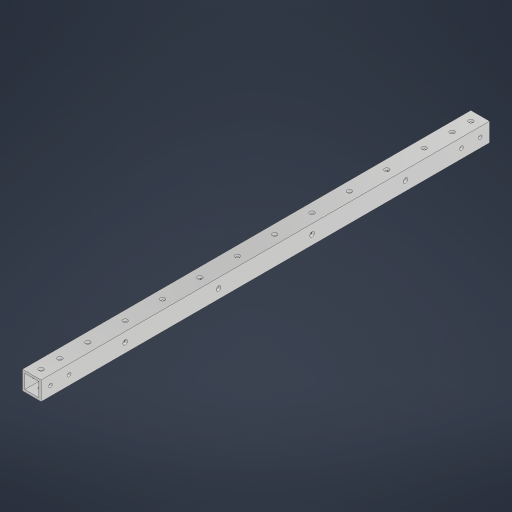
# Autodesk Inventor part: testRoboRescue_Chassis_Frame_widthBar
Saved by Autodesk Inventor 2023 (Build 270158000, 158)
## iProperties
Created: 2022-03-14
Part Number: testRoboRescue_Chassis_Frame_widthBar
Material: Aluminum 6061
Document SubType Name: Modeling
Designer: Nebil Oumer
Density: 2.7 g/cm^3
Appearance: Aluminum - Polished
Mass: 517.114 g
Surface Area: 1215.32 cm^2
Volume: 191.524 cm^3
Author: Nebil Oumer
Autodesk Inventor part; units mm, degrees
ref_plane "YZ Plane" through (0, 0, 0) normal (1, 0, 0) x (0, 1, 0)
ref_plane "XZ Plane" through (0, 0, 0) normal (0, 1, 0) x (-1, 0, 0)
ref_plane "XY Plane" through (0, 0, 0) normal (0, 0, 1) x (1, 0, 0)
sketch "Sketch1" plane through (0, 0, 0) normal (0, 0, 1) x (1, 0, 0)
  line L0 (0, 0) -> (25.4, 0)
  line L1 (25.4, 0) -> (25.4, 25.4)
  line L2 (25.4, 25.4) -> (0, 25.4)
  line L3 (0, 25.4) -> (0, 0)
  line L4 (3.175, 22.225) -> (22.225, 22.225)
  line L5 (22.225, 22.225) -> (22.225, 3.175)
  line L6 (22.225, 3.175) -> (3.175, 3.175)
  line L7 (3.175, 3.175) -> (3.175, 22.225)
  dimension "d0" = 25.4
  dimension "d1" = 25.4
  dimension "d2" = 3.175
  constraints: 16 end point, 4 parallel, 2 perpendicular, 1 horizontal, 3 other
  measures "d0" distance of L2.end L1.end
  measures "d1" distance of L1.end L0.end
  measures "d2" distance between parallel lines of L2 L4
extrude "Extrusion1" add sketch "Sketch1" along normal blind 609.6
sketch "Sketch2" plane through (0, 25.4, 0) normal (0, 1, 0) x (1, 0, 0)
  line L0 (25.4, 0) -> (25.4, -609.6) projected
  line L1 (25.4, -609.6) -> (0, -609.6) projected
  point P0 (0, 0)
  point P1 (12.7, -596.9)
  dimension "d12" = 12.7
  dimension "d13" = 12.7
  measures "d12" distance from line of L0 point (12.7, -596.9)
  measures "d13" distance from line of L1 point (12.7, -596.9)
hole "Hole1" at (12.7, 25.4, 596.9) direction (0, -1, 0) diameter 6.35 end through all
sketch "Sketch3" plane through (0, 25.4, 0) normal (0, 1, 0) x (1, 0, 0)
  line L0 (25.4, 0) -> (0, 0) projected
  line L1 (25.4, 0) -> (25.4, -609.6) projected
  point P0 (12.7, -12.7)
  dimension "d14" = 12.7
  dimension "d15" = 12.7
  measures "d14" distance from line of L0 point (12.7, -12.7)
  measures "d15" distance from line of L1 point (12.7, -12.7)
hole "Hole2" at (12.7, 25.4, 12.7) direction (0, -1, 0) diameter 6.35 end through all
pattern_linear "Rectangular Pattern1" count 2 spacing 25.4 along (0, 0, -1) count 2 spacing 25.4 along (0, 0, 1) of "Hole1", "Hole2"
sketch "Sketch4" plane through (25.4, 0, 0) normal (1, 0, 0) x (0, 0, -1)
  line L0 (0, 25.4) -> (-609.6, 25.4) projected
  line L1 (-609.6, 0) -> (-609.6, 25.4) projected
  line L2 (0, 0) -> (0, 25.4) projected
  point P0 (-596.9, 12.7)
  point P1 (-12.7, 12.7)
  dimension "d29" = 12.7
  dimension "d30" = 12.7
  dimension "d31" = 12.7
  dimension "d32" = 12.7
  measures "d29" distance from line of L0 point (-596.9, 12.7)
  measures "d30" distance from line of L1 point (-596.9, 12.7)
  measures "d31" distance from line of L2 point (-12.7, 12.7)
  measures "d32" distance from line of L0 point (-12.7, 12.7)
hole "Hole3" at (25.4, 12.7, 596.9) at (25.4, 12.7, 12.7) direction (-1, 0, 0) diameter 5.08 end through all
pattern_linear "Rectangular Pattern2" count 2 spacing 25.4 along (0, 0, -1) count 2 spacing 25.4 along (0, 0, 1) of "Hole3"
sketch "Sketch5" plane through (0, 25.4, 0) normal (0, 1, 0) x (1, 0, 0)
  line L0 (25.4, 0) -> (25.4, -609.6) projected
  circle A0 centre (12.7, -571.5) radius 3.175 projected
  point P0 (0, 0)
  point P1 (12.7, -533.4)
  dimension "d46" = 12.7
  dimension "d54" = 38.1
  measures "d46" distance from line of L0 point (12.7, -533.4)
  measures "d54" distance of point (12.7, -533.4) A0.centre
hole "Hole4" at (12.7, 25.4, 533.4) direction (0, -1, 0) diameter 6.35 end through all
pattern_linear "Rectangular Pattern3" count 10 spacing 50.8 along (0, 0, -1) of "Hole4"
sketch "Sketch6" plane through (25.4, 0, 0) normal (1, 0, 0) x (0, 0, -1)
  line L0 (0, 25.4) -> (-609.6, 25.4) projected
  line L1 (-609.6, 0) -> (-609.6, 25.4) projected
  point P0 (0, 0)
  point P1 (-495.3, 12.7)
  dimension "d58" = 12.7
  dimension "d66" = 114.3
  measures "d58" distance from line of L0 point (-495.3, 12.7)
  measures "d66" distance from line of L1 point (-495.3, 12.7)
hole "Hole5" at (25.4, 12.7, 495.3) direction (-1, 0, 0) diameter 6.35 end through all
pattern_linear "Rectangular Pattern4" count 4 spacing 127 along (0, 0, -1) of "Hole5"
equation "\"d0\" = d1"
body "Solid1"
